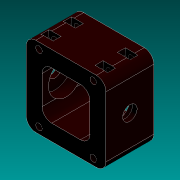
# Autodesk Inventor part: gearbox v2 mid part
Saved by Autodesk Inventor 2020 (Build 240168000, 168)
## iProperties
Created: 2020-05-25
Part Number: gearbox v2 mid part
Material: ABS Plastic
Document SubType Name: Modeling
Designer: stefa
Density: 1.06 g/cm^3
Appearance: Default
Author: stefa
Autodesk Inventor part; units mm, degrees
ref_plane "YZ Plane" through (0, 0, 0) normal (1, 0, 0) x (0, 1, 0)
ref_plane "XZ Plane" through (0, 0, 0) normal (0, 1, 0) x (-1, 0, 0)
ref_plane "XY Plane" through (0, 0, 0) normal (0, 0, 1) x (1, 0, 0)
sketch "Sketch1" plane through (0, 0, 0) normal (0, 0, 1) x (1, 0, 0)
  line L0 (-25, -25) -> (25, -25)
  line L1 (25, -25) -> (25, 25)
  line L2 (25, 25) -> (-25, 25)
  line L3 (-25, 25) -> (-25, -25)
  line L4 (-25, -25) -> (25, 25) construction
  line L5 (25, -25) -> (-25, 25) construction
  line L6 (-15, 15) -> (15, 15)
  line L7 (15, 15) -> (15, -15)
  line L8 (15, -15) -> (-15, -15)
  line L9 (-15, -15) -> (-15, 15)
  point P0 (0, 0)
  dimension "d0" = 50
  dimension "d1" = 50
  dimension "d2" = 10
  constraints: 20 end point, 4 parallel, 2 midpoint, 2 perpendicular, 1 horizontal, 3 other
  measures "d0" distance of L2.end L1.end
  measures "d1" distance of L1.end L0.end
  measures "d2" distance between parallel lines of L2 L6
extrude "Extrusion1" add sketch "Sketch1" along normal mid plane 30
sketch "Sketch2" plane through (-15, -15, 15) normal (1, 0, 0) x (0, 0, -1)
  circle A0 centre (15, 15) radius 11
  circle A1 centre (15, 15) radius 4.5
  line L0 (30, 40) -> (0, 40) projected
  line L1 (30, -10) -> (0, -10) projected
  line L2 (30, 40) -> (30, -10) projected
  dimension "d5" = 22
  dimension "d6" = 9
  dimension "d7" = 25
  dimension "d8" = 50
  dimension "d9" = 15
  constraints: 2 centre point, 1 coincident
  measures "d5" diameter of A0
  measures "d6" diameter of A1
  measures "d7" distance from line of L0 A0.centre
  measures "d8" distance between parallel lines of L1 L0
  measures "d9" distance from line of L2 A0.centre
extrude "Extrusion2" cut sketch "Sketch2" against normal blind 7
extrude "Extrusion3" cut sketch "Sketch2" against normal through all contours A1
mirror "Mirror1" about plane through (0, 0, 0) normal (1, 0, 0) of "Extrusion2", "Extrusion3"
ref_plane "Work Plane1" through (0, 0, 10) normal (0, 0, 1) x (1, 0, 0)
sketch "Sketch6" plane through (0, 0, 10) normal (0, 0, 1) x (1, 0, 0)
  line L0 (-18.9197, -24.325) -> (-20.8394, -21)
  line L1 (-20.8394, -21) -> (-18.9197, -17.675)
  line L2 (-18.9197, -17.675) -> (-15.0803, -17.675)
  line L3 (-15.0803, -17.675) -> (-13.1606, -21)
  line L4 (-13.1606, -21) -> (-15.0803, -24.325)
  line L5 (-15.0803, -24.325) -> (-18.9197, -24.325)
  line L6 (-25, -25) -> (25, -25) projected
  line L7 (-25, 25) -> (-25, -25) projected
  line L8 (-13.1606, -21) -> (-13.1606, -25)
  line L9 (-20.8394, -21) -> (-20.8394, -25)
  point P0 (0, 0)
  point P1 (-17, -21)
  dimension "d18" = 8
  dimension "d19" = 4
  dimension "d20" = 6.65
  constraints: 16 end point, 2 point on line, 1 parallel, 1 perpendicular, 1 vertical, 13 other
  measures "d18" distance from line of L7 point (-17, -21)
  measures "d19" distance from line of point (-17, -21) L6
  measures "d20" distance between parallel lines of L2 L5
extrude "Extrusion4" cut sketch "Sketch6" against normal blind 5
pattern_linear "Rectangular Pattern1" count 2 spacing 34 along (1, 0, 0) count 2 spacing 14 along (0, 0, -1) of "Extrusion4"
sketch "Sketch7" plane through (0, 0, 15) normal (0, 0, 1) x (1, 0, 0)
  circle A0 centre (-17, -21) radius 2
  line L0 (-25, 25) -> (-25, -25) projected
  line L1 (-25, -25) -> (25, -25) projected
  point P0 (0, 0)
  dimension "d29" = 4
  dimension "d30" = 8
  dimension "d31" = 4
  constraints: 1 centre point
  measures "d29" diameter of A0
  measures "d30" distance from line of L0 A0.centre
  measures "d31" distance from line of L1 A0.centre
extrude "Extrusion5" cut sketch "Sketch7" against normal through all
pattern_linear "Rectangular Pattern2" count 2 spacing 34 along (1, 0, 0) of "Extrusion5"
mirror "Mirror3" about plane through (0, 0, 0) normal (0, 1, 0) of "Extrusion4", "Rectangular Pattern1", "Extrusion5", "Rectangular Pattern2"
fillet "Fillet1" radius 6 8 edges at (-25, 25, 0) (-25, -25, 0) (25, -25, 0) (25, 25, 0) (15, 15, 0) (-15, 15, 0) (15, -15, 0) (-15, -15, 0)
equation "\"d7\" = 0.5 * d8"
body "Solid1"
